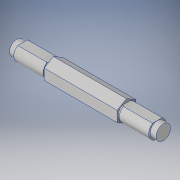
# Autodesk Inventor part: Flywheel Axle
Saved by Autodesk Inventor 2019.4 (Build 234330000, 330)
## iProperties
Created: 2020-01-12
Part Number: Flywheel Axle
Material: Aluminum 6061
Document SubType Name: Modeling
Designer: admin
Density: 2.7 g/cm^3
Appearance: Aluminum - Flat
Author: admin
Autodesk Inventor part; units mm, degrees
ref_plane "YZ Plane" through (0, 0, 0) normal (1, 0, 0) x (0, 1, 0)
ref_plane "XZ Plane" through (0, 0, 0) normal (0, 1, 0) x (-1, 0, 0)
ref_plane "XY Plane" through (0, 0, 0) normal (0, 0, 1) x (1, 0, 0)
sketch "Sketch1" plane through (0, 0, 0) normal (0, 0, 1) x (1, 0, 0)
  line L0 (0, 0) -> (0, 5)
  line L1 (0, 5) -> (4, 5)
  line L2 (4, 5) -> (4, 6)
  line L3 (96.4, 6) -> (96.4, 5)
  line L4 (96.4, 5) -> (100.4, 5)
  line L5 (100.4, 5) -> (100.4, 0)
  line L6 (100.4, 0) -> (0, 0)
  line L7 (4, 6) -> (25.2, 6)
  line L8 (25.2, 6) -> (25.2, 8)
  line L9 (25.2, 8) -> (75.2, 8)
  line L10 (75.2, 8) -> (75.2, 6)
  line L11 (75.2, 6) -> (96.4, 6)
  dimension "d1" = 5
  dimension "d2" = 4
  dimension "d3" = 4
  dimension "d4" = 92.4
  dimension "d5" = 2
  dimension "d6" = 50
  dimension "d7" = 6
  constraints: 24 end point, 9 perpendicular, 3 point on line, 1 collinear, 1 horizontal, 1 vertical
  measures "d1" distance between parallel lines of L6 L1
  measures "d2" distance of L0.end L1.end
  measures "d3" distance of L3.end L4.end
  measures "d4" distance of L2.end L3.start
  measures "d5" distance of L7.end L8.end
  measures "d6" distance of L8.end L9.end
  measures "d7" distance between parallel lines of L6 L7
revolve "Revolution1" add sketch "Sketch1" angle 360 about axis through (100.4, 0, 0) along (-1, 0, 0)
sketch "Sketch2" plane through (25.2, 0, 0) normal (-1, 0, 0) x (0, 0, 1)
  line L0 (0, 7.3323) -> (6.35, 3.6662)
  line L1 (6.35, 3.6662) -> (6.35, -3.6662)
  line L2 (6.35, -3.6662) -> (0, -7.3323)
  line L3 (0, -7.3323) -> (-6.35, -3.6662)
  line L4 (-6.35, -3.6662) -> (-6.35, 3.6662)
  line L5 (-6.35, 3.6662) -> (0, 7.3323)
  circle A0 centre (0, 0) radius 8 projected
  dimension "d9" = 12.7
  constraints: 12 end point, 1 coincident, 13 other
  measures "d9" distance between parallel lines of L4 L1
extrude "Extrusion1" cut sketch "Sketch2" against normal through all
sketch "Sketch4" plane through (25.2, -3.6662, -6.35) normal (-1, 0, 0) x (0, 0, 1)
  circle A0 centre (6.35, 3.6662) radius 5 projected
  circle A1 centre (6.35, 3.6662) radius 5.75
  circle A2 centre (6.35, 3.6662) radius 6 projected
  dimension "d14" = 11.5
  constraints: 1 centre point, 1 coincident
  measures "d14" diameter of A1
extrude "Extrusion3" cut sketch "Sketch4" along normal blind 1.1 contours A2
sketch "Sketch3" plane through (4, 0, 0) normal (-1, 0, 0) x (0, 0, 1)
  line L0 (-3.3166, 5) -> (3.3166, 5)
  circle A0 centre (0, 0) radius 5 projected
  circle A1 centre (0, 0) radius 6 projected
  constraints: 2 end point, 2 point on circle, 1 horizontal, 1 tangent
extrude "Extrusion2" cut sketch "Sketch3" against normal up to surface (21.2 mm away) contours A1 L0 picked at (1.794, 5.2111)
ref_plane "Work Plane1" through (50.2, -3.6662, 6.35) normal (1, 0, 0) x (0, 0, -1)
mirror "Mirror1" about plane through (50.2, -3.6662, 6.35) normal (1, 0, 0) of "Extrusion3", "Extrusion2"
body "Solid1"
